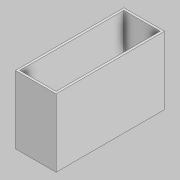
# Autodesk Inventor part: GameDesignBox
Saved by Autodesk Inventor 2021 (Build 250183000, 183)
## iProperties
Created: 2021-03-03
Part Number: GameDesignBox
Material: Generic
Document SubType Name: Modeling
Designer: Merkileg
Density: 1 g/cm^3
Appearance: Default
Author: Merkileg
Autodesk Inventor part; units mm, degrees
ref_plane "YZ Plane" through (0, 0, 0) normal (1, 0, 0) x (0, 1, 0)
ref_plane "XZ Plane" through (0, 0, 0) normal (0, 1, 0) x (-1, 0, 0)
ref_plane "XY Plane" through (0, 0, 0) normal (0, 0, 1) x (1, 0, 0)
sketch "Sketch1" plane through (0, 0, 0) normal (0, 1, 0) x (-1, 0, 0)
  line L0 (0, 0) -> (457.2, 0)
  line L1 (457.2, 0) -> (457.2, -1219.2)
  line L2 (457.2, -1219.2) -> (0, -1219.2)
  line L3 (0, -1219.2) -> (0, 0)
  line L4 (25.4, -25.4) -> (431.8, -25.4)
  line L5 (431.8, -25.4) -> (431.8, -1193.8)
  line L6 (431.8, -1193.8) -> (25.4, -1193.8)
  line L7 (25.4, -1193.8) -> (25.4, -25.4)
  dimension "d0" = 457.2
  dimension "d1" = 1219.2
  dimension "d2" = 25.4
  dimension "d3" = 25.4
  dimension "d4" = 25.4
  dimension "d5" = 25.4
  constraints: 16 end point, 4 parallel, 2 horizontal, 2 perpendicular
  measures "d0" distance of L1.end L2.end
  measures "d1" distance of L0.end L1.end
  measures "d2" distance between parallel lines of L1 L5
  measures "d3" distance between parallel lines of L0 L4
  measures "d4" distance between parallel lines of L7 L3
  measures "d5" distance between parallel lines of L2 L6
extrude "Extrusion1" add sketch "Sketch1" along normal blind 762
sketch "Sketch2" plane through (0, 0, 0) normal (0, -1, 0) x (1, 0, 0)
  line L0 (-25.4, -25.4) -> (-431.8, -25.4) projected
  line L1 (-431.8, -1193.8) -> (-25.4, -1193.8) projected
  line L2 (-431.8, -25.4) -> (-25.4, -25.4)
  line L3 (-25.4, -25.4) -> (-25.4, -1193.8)
  line L4 (-25.4, -1193.8) -> (-431.8, -1193.8)
  line L5 (-431.8, -1193.8) -> (-431.8, -25.4)
  point P0 (0, 0)
  constraints: 8 end point, 2 parallel, 1 horizontal, 1 perpendicular
extrude "Extrusion2" add sketch "Sketch2" against normal blind 25.4
body "Solid1"
